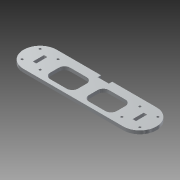
# Autodesk Inventor part: OpenROV 2_3 Dev Horizontal Motor Mount
Saved by Autodesk Inventor 2015 (Build 190159000, 159)
## iProperties
Created: 2011-11-06
Part Number: OpenROV 2_3 Dev Horizontal Motor Mount
Document SubType Name: Modeling
Designer: user
Density: 1 g/cm^3
Material: Generic
Appearance: Default
Author: user
Autodesk Inventor part; units mm, degrees
ref_plane "YZ Plane" through (0, 0, 0) normal (1, 0, 0) x (0, 1, 0)
ref_plane "XZ Plane" through (0, 0, 0) normal (0, 1, 0) x (-1, 0, 0)
ref_plane "XY Plane" through (0, 0, 0) normal (0, 0, 1) x (1, 0, 0)
sketch "Sketch1" plane through (0, 0, 0) normal (0, 0, 1) x (1, 0, 0)
  line L0 (120, -15) -> (120, -15)
  line L1 (105, -30) -> (15, -30)
  line L2 (0, -15) -> (0, -15)
  line L3 (13.5, -10) -> (16.5, -10)
  line L4 (16.5, -10) -> (16.5, -20)
  line L5 (16.5, -20) -> (13.5, -20)
  line L6 (13.5, -20) -> (13.5, -10)
  line L7 (103.5, -10) -> (106.5, -10)
  line L8 (106.5, -10) -> (106.5, -20)
  line L9 (106.5, -20) -> (103.5, -20)
  line L10 (103.5, -20) -> (103.5, -10)
  arc A0 (15, 0) -> (0, -15) centre (15, -15) ccw
  arc A1 (0, -15) -> (15, -30) centre (15, -15) ccw
  arc A2 (105, -30) -> (120, -15) centre (105, -15) ccw
  arc A3 (120, -15) -> (105, 0) centre (105, -15) ccw
  line L11 (65, 0) -> (65, -3)
  line L12 (65, -3) -> (55, -3)
  line L13 (55, -3) -> (55, 0)
  line L14 (15, 0) -> (55, 0)
  line L15 (65, 0) -> (105, 0)
  line L16 (90, -13) -> (90, -21)
  line L17 (30, -21) -> (30, -13)
  arc A4 (35, -8) -> (30, -13) centre (35, -13) ccw
  arc A5 (90, -13) -> (85, -8) centre (85, -13) ccw
  arc A6 (85, -26) -> (90, -21) centre (85, -21) ccw
  arc A7 (30, -21) -> (35, -26) centre (35, -21) ccw
  line L18 (65, -13) -> (65, -21)
  line L19 (55, -21) -> (55, -13)
  line L20 (35, -8) -> (50, -8)
  line L21 (70, -8) -> (85, -8)
  line L22 (85, -26) -> (70, -26)
  line L23 (50, -26) -> (35, -26)
  arc A8 (55, -13) -> (50, -8) centre (50, -13) ccw
  arc A9 (50, -26) -> (55, -21) centre (50, -21) ccw
  arc A10 (65, -21) -> (70, -26) centre (70, -21) ccw
  arc A11 (70, -8) -> (65, -13) centre (70, -13) ccw
  circle A12 centre (6.868, -6.868) radius 1
  circle A13 centre (6.868, -23.132) radius 1
  circle A14 centre (23.132, -23.132) radius 1
  circle A15 centre (23.132, -6.868) radius 1
  circle A16 centre (113.132, -6.868) radius 1
  circle A17 centre (96.868, -6.868) radius 1
  circle A18 centre (96.868, -23.132) radius 1
  circle A19 centre (113.132, -23.132) radius 1
  point P0 (0, 0)
  point P1 (120, 0)
  point P2 (0, -30)
  dimension "d0" = 30
  dimension "d1" = 120
  dimension "d2" = 10
  dimension "d3" = 3
  dimension "d4" = 13.5
  dimension "d5" = 10
  dimension "d6" = 87
  dimension "d7" = 3
  dimension "d8" = 10
  dimension "d9" = 10
  dimension "d10" = 15
  dimension "d11" = 10
  dimension "d12" = 55
  dimension "d13" = 3
  dimension "d18" = 30
  dimension "d19" = 30
  dimension "d20" = 5
  dimension "d23" = 25
  dimension "d24" = 25
  dimension "d25" = 5
  dimension "d27" = 8
  dimension "d30" = 2
  dimension "d31" = 8.132
  dimension "d32" = 8.132
  dimension "d35" = 360
  dimension "d37" = 2
  dimension "d40" = 8.132
  dimension "d41" = 8.132
  dimension "d44" = 360
  dimension "d48" = 18
  dimension "d50" = 3
  dimension "d51" = 15
  constraints: 48 end point, 30 tangent, 24 point on circle, 20 centre point, 14 parallel, 9 equal radius, 6 horizontal, 6 perpendicular, 4 point on line, 18 other
  measures "d0" distance of point (0, -30) point (0, 0)
  measures "d1" distance of point (0, 0) point (120, 0)
  measures "d2" distance of L5.end L3.start
  measures "d3" distance of L3.start L3.end
  measures "d4" distance between parallel lines of L2 L6
  measures "d5" distance between parallel lines of L1 L5
  measures "d6" distance between parallel lines of L4 L10
  measures "d7" distance of L7.start L7.end
  measures "d8" distance of L7.end L8.end
  measures "d9" distance between parallel lines of L1 L9
  measures "d10" radius of A0
  measures "d11" distance of L11.end L12.end
  measures "d12" distance from line of L2.end L13
  measures "d13" distance of L11.start L11.end
  measures "d18" distance from line of L0.start L16
  measures "d19" distance from line of L2.start L17
  measures "d20" radius of A4
  measures "d23" distance between parallel lines of L17 L19
  measures "d24" distance between parallel lines of L16 L18
  measures "d25" radius of A8
  measures "d27" distance between parallel lines of L15 L21
  measures "d30" diameter of A12
  measures "d31" horizontal distance of A1.centre A12.centre
  measures "d32" horizontal distance of A1.centre A12.centre
  measures "d37" diameter of A16
  measures "d40" horizontal distance of A2.centre A16.centre
  measures "d41" horizontal distance of A2.centre A16.centre
  measures "d48" distance between parallel lines of L23 L20
  measures "d50" distance from line of point (0, 0) L12
  measures "d51" horizontal distance of A0.centre point (0, 0)
extrude "Extrusion4" add sketch "Sketch1" along normal blind 3
body "Solid4"
